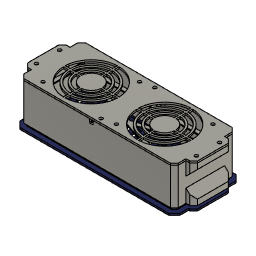
Exhaust (Autodesk Fusion 360 archive; units mm, degrees)
design "Exhaust Fan Cover"
Autodesk Fusion 360 part; units mm, degrees
(part 1 of 2)
sketch "Skizze1" plane through (0, 0, 0) normal (0, 0, 1) x (1, 0, 0)
  line L0 (0, 0) -> (160, 0)
  line L1 (160, 0) -> (160, 64)
  line L2 (160, 64) -> (0, 64)
  line L3 (0, 64) -> (0, 0)
  dimension "d1" = 160
  dimension "d2" = 64
  constraint horizontal L0
  constraint vertical L1
  constraint horizontal L2
  constraint vertical L3
  constraint coincident L0.start L3.end
  measures "d1" distance of L0.start L0.end
  measures "d2" distance of L0.start L2.end
extrude "Extrusion1" add sketch "Skizze1" along normal blind 40 makes body 1
chamfer "Fase1" distance 4 angle 45 4 edges at (160, 0, 20) (160, 64, 20) (0, 0, 20) (0, 64, 20) on bodies 1
shell "Schale1" thickness 1.8 removed faces 1 at (54.6667, 42.6667, 40) on bodies 1
sketch "Skizze2" plane through (0, 0, 1.8) normal (0, 0, 1) x (-1, 0, 0)
  line L0 (-4.7456, -62.2) -> (-1.8, -59.2544)
  line L1 (-1.8, -59.2544) -> (-1.8, -4.7456)
  line L2 (-1.8, -4.7456) -> (-4.7456, -1.8)
  line L3 (-4.7456, -1.8) -> (-155.2544, -1.8)
  line L4 (-155.2544, -1.8) -> (-158.2, -4.7456)
  line L5 (-158.2, -4.7456) -> (-158.2, -59.2544)
  line L6 (-158.2, -59.2544) -> (-155.2544, -62.2)
  line L7 (-155.2544, -62.2) -> (-4.7456, -62.2)
  line L8 (-80, -57) -> (-80, -7) construction
  line L9 (-78, -7) -> (-69.1837, -57)
  line L10 (-69.1837, -57) -> (-65.1219, -57)
  line L11 (-65.1219, -57) -> (-73.9383, -7)
  line L12 (-73.9383, -7) -> (-78, -7)
  line L13 (-56.8362, -57) -> (-65.6526, -7)
  line L14 (-69.7143, -7) -> (-60.8979, -57)
  line L15 (-60.8979, -57) -> (-56.8362, -57)
  line L16 (-65.6526, -7) -> (-69.7143, -7)
  line L17 (-48.5505, -57) -> (-57.3669, -7)
  line L18 (-61.4286, -7) -> (-52.6122, -57)
  line L19 (-52.6122, -57) -> (-48.5505, -57)
  line L20 (-57.3669, -7) -> (-61.4286, -7)
  line L21 (-40.2648, -57) -> (-49.0812, -7)
  line L22 (-53.1429, -7) -> (-44.3265, -57)
  line L23 (-44.3265, -57) -> (-40.2648, -57)
  line L24 (-49.0812, -7) -> (-53.1429, -7)
  line L25 (-31.9791, -57) -> (-40.7954, -7)
  line L26 (-44.8571, -7) -> (-36.0408, -57)
  line L27 (-36.0408, -57) -> (-31.9791, -57)
  line L28 (-40.7954, -7) -> (-44.8571, -7)
  line L29 (-23.6934, -57) -> (-32.5097, -7)
  line L30 (-36.5714, -7) -> (-27.7551, -57)
  line L31 (-27.7551, -57) -> (-23.6934, -57)
  line L32 (-32.5097, -7) -> (-36.5714, -7)
  line L33 (-15.4077, -57) -> (-24.224, -7)
  line L34 (-28.2857, -7) -> (-19.4694, -57)
  line L35 (-19.4694, -57) -> (-15.4077, -57)
  line L36 (-24.224, -7) -> (-28.2857, -7)
  line L37 (-7.1219, -57) -> (-15.9383, -7)
  line L38 (-20, -7) -> (-11.1837, -57)
  line L39 (-11.1837, -57) -> (-7.1219, -57)
  line L40 (-15.9383, -7) -> (-20, -7)
  line L41 (-11.7183, -7) -> (-8, -28.0875)
  line L42 (-11.7183, -7) -> (13.942, -7) construction
  line L43 (-8, -28.0875) -> (-7, -28.0875)
  line L44 (-7, -10.7237) -> (-7.6566, -7)
  line L45 (-7.6566, -7) -> (-11.7183, -7)
  line L46 (-7, -28.0875) -> (-7, -10.7237)
  line L47 (-119.7352, -57) -> (-110.9188, -7)
  line L48 (-153, -28.0875) -> (-153, -10.7237)
  line L49 (-152, -28.0875) -> (-153, -28.0875)
  line L50 (-98.5714, -7) -> (-107.3878, -57)
  line L51 (-152.3434, -7) -> (-148.2817, -7)
  line L52 (-119.2046, -7) -> (-115.1429, -7)
  line L53 (-132.2449, -57) -> (-136.3066, -57)
  line L54 (-135.776, -7) -> (-131.7143, -7)
  line L55 (-140.5306, -57) -> (-144.5923, -57)
  line L56 (-102.6331, -7) -> (-98.5714, -7)
  line L57 (-153, -10.7237) -> (-152.3434, -7)
  line L58 (-99.1021, -57) -> (-103.1638, -57)
  line L59 (-106.8571, -7) -> (-115.6735, -57)
  line L60 (-107.3878, -57) -> (-111.4495, -57)
  line L61 (-123.9592, -57) -> (-128.0209, -57)
  line L62 (-115.6735, -57) -> (-119.7352, -57)
  line L63 (-128.0209, -57) -> (-119.2046, -7)
  line L64 (-144.5923, -57) -> (-135.776, -7)
  line L65 (-111.4495, -57) -> (-102.6331, -7)
  line L66 (-131.7143, -7) -> (-140.5306, -57)
  line L67 (-148.8163, -57) -> (-152.8781, -57)
  line L68 (-123.4286, -7) -> (-132.2449, -57)
  line L69 (-140, -7) -> (-148.8163, -57)
  line L70 (-148.2817, -7) -> (-152, -28.0875)
  line L71 (-115.1429, -7) -> (-123.9592, -57)
  line L72 (-127.4903, -7) -> (-123.4286, -7)
  line L73 (-144.0617, -7) -> (-140, -7)
  line L74 (-90.8163, -57) -> (-94.8781, -57)
  line L75 (-90.2857, -7) -> (-99.1021, -57)
  line L76 (-82, -7) -> (-90.8163, -57)
  line L77 (-86.0617, -7) -> (-82, -7)
  line L78 (-103.1638, -57) -> (-94.3474, -7)
  line L79 (-94.3474, -7) -> (-90.2857, -7)
  line L80 (-110.9188, -7) -> (-106.8571, -7)
  line L81 (-94.8781, -57) -> (-86.0617, -7)
  line L82 (-136.3066, -57) -> (-127.4903, -7)
  line L83 (-152.8781, -57) -> (-144.0617, -7)
  line L84 (-78.7624, -26.609) -> (-73.4037, -57)
  line L85 (-73.4037, -57) -> (-77.4654, -57)
  line L86 (-77.4654, -57) -> (-79.1, -47.7295)
  line L87 (-79.1, -47.7295) -> (-80, -47.7295)
  line L88 (-78.7624, -26.609) -> (-80, -26.609)
  line L89 (-82.5346, -57) -> (-80.9, -47.7295)
  line L90 (-86.5963, -57) -> (-82.5346, -57)
  line L91 (-81.2376, -26.609) -> (-86.5963, -57)
  line L92 (-81.2376, -26.609) -> (-80, -26.609)
  line L93 (-80.9, -47.7295) -> (-80, -47.7295)
  line L94 (-7, -57) -> (-7, -7) construction
  line L95 (-7, -7) -> (-153, -7) construction
  line L96 (-153, -7) -> (-153, -57) construction
  line L97 (-153, -57) -> (-7, -57) construction
  point P0 (-80, -57)
  point P1 (-80, -7)
  dimension "d7" = -5.2
  dimension "d8" = 4
  dimension "d9" = 80
  dimension "d10" = 2
  dimension "d13" = 58
  dimension "d14" = 0
  dimension "d15" = 80
  dimension "d16" = 4
  dimension "d17" = 4.22
  dimension "d18" = 1
  dimension "d19" = 4
  dimension "d20" = 0.9
  dimension "d21" = 4.22
  constraint midpoint P0 L97
  constraint midpoint P1 L95
  constraint coincident L9.start L95
  constraint coincident L9.end L97
  constraint coincident L10.end L97
  constraint coincident L11.end L95
  constraint parallel L9 L11
  constraint horizontal L42
  constraint coincident L41.start L95
  constraint coincident L44.start L94
  constraint perpendicular L43 L94
  constraint parallel L41 L44
  constraint coincident L44.end L95
  constraint coincident L43.end L94
  constraint symmetric P0 L8 L8.start
  constraint symmetric P1 L8 L8.end
  constraint symmetric L8 L9.start L76.start
  constraint symmetric L8 L9.end L74.start
  constraint symmetric L8 L10.end L74.end
  constraint symmetric L8 L11.end L77.start
  constraint symmetric L8 L13.start L58.end
  constraint symmetric L8 L13.end L78.end
  constraint symmetric L8 L14.start L75.start
  constraint symmetric L8 L14.end L58.start
  constraint symmetric L8 L17.start L60.end
  constraint symmetric L8 L17.end L56.start
  constraint symmetric L8 L18.start L50.start
  constraint symmetric L8 L18.end L50.end
  constraint symmetric L8 L21.start L47.start
  constraint symmetric L8 L21.end L47.end
  constraint symmetric L8 L22.start L59.start
  constraint symmetric L8 L22.end L59.end
  constraint symmetric L8 L25.start L61.end
  constraint symmetric L8 L25.end L52.start
  constraint symmetric L8 L26.start L52.end
  constraint symmetric L8 L26.end L61.start
  constraint symmetric L8 L29.start L53.end
  constraint symmetric L8 L29.end L72.start
  constraint symmetric L8 L30.start L68.start
  constraint symmetric L8 L30.end L53.start
  constraint symmetric L8 L33.start L55.end
  constraint symmetric L8 L33.end L54.start
  constraint symmetric L8 L34.start L54.end
  constraint symmetric L8 L34.end L55.start
  constraint symmetric L8 L37.start L67.end
  constraint symmetric L8 L37.end L73.start
  constraint symmetric L8 L38.start L69.start
  constraint symmetric L8 L38.end L67.start
  constraint symmetric L8 L41.start L51.end
  constraint symmetric L8 L41.end L49.start
  constraint symmetric L8 L44.start L48.end
  constraint symmetric L8 L44.end L51.start
  constraint symmetric L8 L43.end L48.start
  constraint coincident L84.end L97
  constraint parallel L9 L84
  constraint coincident L85.end L97
  constraint parallel L84 L86
  constraint coincident L8 L87.end
  constraint perpendicular L8 L87
  constraint coincident L8 L88.end
  constraint perpendicular L8 L88
  constraint symmetric L8 L84.start L91.start
  constraint symmetric L8 L84.end L90.start
  constraint symmetric L8 L85.end L89.start
  constraint symmetric L8 L86.end L89.end
  constraint symmetric L8 L87.end L93.end
  constraint symmetric L8 L88.end L92.end
  measures "d8" distance of L9 L11
  measures "d9" angle of L11 L95
  measures "d10" distance of P1 L9.start
  measures "d15" angle of L41 L42
  measures "d16" distance of L41 L44
  measures "d17" distance of L37.end L41.start
  measures "d18" distance of L41.end L43.end
  measures "d19" distance of L84 L86
  measures "d20" distance of L86.end L87.end
  measures "d21" distance of L9.end L84.end
extrude "Extrusion2" cut sketch "Skizze2" against normal blind 1.8 contours L9 L10 L11 L12 | L13 L14 L15 L16 | L17 L18 L19 L20 | L21 L22 L23 L24 | L25 L26 L27 L28 | L29 L30 L31 L32 | L33 L34 L35 L36 | L37 L38 L39 L40 | L41 L43 L44 L45 L46 | L47 L59 L62 L80 | L48 L49 L51 L57 L70 | L50 L56 L60 L65 | L52 L61 L63 L71 | L53 L68 L72 L82 | L54 L55 L64 L66 | L58 L75 L78 L79 | L67 L69 L73 L83 | L74 L76 L77 L81 | L84 L85 L86 L87 L88 L89 L90 L91 L92 L93 bodies 1
ref_plane "Arbeitsebene1" through (80, 32, 1.8) normal (0, 0, -1) x (-1, 0, 0)
split "Teilen1" by plane through (80, 32, 1.8) normal (0, 0, -1) bodies 1 makes body 2 at (80.6667, 2.3333, 0)
sketch "Skizze3" plane through (0, 0, 1.8) normal (0, 0, -1) x (1, 0, 0)
  line L0 (158.2, -59.2544) -> (155.2544, -62.2)
  line L1 (155.2544, -62.2) -> (4.7456, -62.2)
  line L2 (4.7456, -62.2) -> (1.8, -59.2544)
  line L3 (1.8, -59.2544) -> (1.8, -4.7456)
  line L4 (1.8, -4.7456) -> (4.7456, -1.8)
  line L5 (4.7456, -1.8) -> (155.2544, -1.8)
  line L6 (155.2544, -1.8) -> (158.2, -4.7456)
  line L7 (158.2, -4.7456) -> (158.2, -59.2544)
  line L8 (156, -64) -> (160, -60)
  line L9 (160, -60) -> (160, -4)
  line L10 (160, -4) -> (156, 0)
  line L11 (156, 0) -> (4, 0)
  line L12 (4, 0) -> (0, -4)
  line L13 (0, -4) -> (0, -60)
  line L14 (0, -60) -> (4, -64)
  line L15 (4, -64) -> (156, -64)
  line L16 (80, -1.8) -> (80, -62.2) construction
  line L17 (0, -12) -> (-8, -12)
  line L18 (-8, -12) -> (-8, -52)
  line L19 (-8, -52) -> (0, -52)
  line L20 (0, -52) -> (0, -12)
  line L21 (80, -32) -> (1.8, -32) construction
  line L22 (160, -12) -> (168, -12)
  line L23 (168, -12) -> (168, -52)
  line L24 (168, -52) -> (160, -52)
  dimension "d25" = 40
  dimension "d26" = 8
  constraint midpoint L5 L16.start
  constraint midpoint L1 L16.end
  constraint horizontal L17
  constraint vertical L18
  constraint horizontal L19
  constraint vertical L20
  constraint coincident L13 L17.start
  constraint midpoint L16 L21.start
  constraint midpoint L3 L21.end
  constraint symmetric L17 L19 L21
  constraint symmetric L16 L17.start L22.start
  constraint symmetric L16 L17.end L22.end
  constraint symmetric L16 L18.end L23.end
  constraint symmetric L16 L19.end L24.end
  measures "d25" distance of L17.end L18.end
  measures "d26" distance of L17.start L17.end
extrude "Extrusion3" add sketch "Skizze3" against normal blind 5.8 contours L9 L22 L23 L24 | L13 L17 L18 L19 L20 bodies 1 2
chamfer "Fase2" distance 4 angle 45 4 edges at (168, 52, 4.7) (168, 12, 4.7) (-8, 52, 4.7) (-8, 12, 4.7) on bodies 1
sketch "Skizze4" plane through (0, 0, 0) normal (0, 0, -1) x (1, 0, 0)
  line L0 (135.776, -7) -> (144.5923, -57)
  line L1 (144.5923, -57) -> (140.5306, -57)
  line L2 (140.5306, -57) -> (131.7143, -7)
  line L3 (131.7143, -7) -> (135.776, -7)
  line L4 (107.3878, -57) -> (98.5714, -7)
  line L5 (98.5714, -7) -> (102.6331, -7)
  line L6 (102.6331, -7) -> (111.4495, -57)
  line L7 (111.4495, -57) -> (107.3878, -57)
  line L8 (78, -7) -> (69.1837, -57)
  line L9 (69.1837, -57) -> (65.1219, -57)
  line L10 (65.1219, -57) -> (73.9383, -7)
  line L11 (73.9383, -7) -> (78, -7)
  line L12 (44.8571, -7) -> (36.0408, -57)
  line L13 (36.0408, -57) -> (31.9791, -57)
  line L14 (31.9791, -57) -> (40.7954, -7)
  line L15 (40.7954, -7) -> (44.8571, -7)
  line L16 (7, -10.7237) -> (7.6566, -7)
  line L17 (7.6566, -7) -> (11.7183, -7)
  line L18 (11.7183, -7) -> (8, -28.0875)
  line L19 (8, -28.0875) -> (7, -28.0875)
  line L20 (7, -28.0875) -> (7, -10.7237)
  line L21 (36.5714, -7) -> (27.7551, -57)
  line L22 (27.7551, -57) -> (23.6934, -57)
  line L23 (23.6934, -57) -> (32.5097, -7)
  line L24 (32.5097, -7) -> (36.5714, -7)
  line L25 (69.7143, -7) -> (60.8979, -57)
  line L26 (60.8979, -57) -> (56.8362, -57)
  line L27 (56.8362, -57) -> (65.6526, -7)
  line L28 (65.6526, -7) -> (69.7143, -7)
  line L29 (103.1638, -57) -> (99.1021, -57)
  line L30 (99.1021, -57) -> (90.2857, -7)
  line L31 (90.2857, -7) -> (94.3474, -7)
  line L32 (94.3474, -7) -> (103.1638, -57)
  line L33 (132.2449, -57) -> (123.4286, -7)
  line L34 (123.4286, -7) -> (127.4903, -7)
  line L35 (127.4903, -7) -> (136.3066, -57)
  line L36 (136.3066, -57) -> (132.2449, -57)
  line L37 (148.8163, -57) -> (140, -7)
  line L38 (140, -7) -> (144.0617, -7)
  line L39 (144.0617, -7) -> (152.8781, -57)
  line L40 (152.8781, -57) -> (148.8163, -57)
  line L41 (119.7352, -57) -> (115.6735, -57)
  line L42 (115.6735, -57) -> (106.8571, -7)
  line L43 (106.8571, -7) -> (110.9188, -7)
  line L44 (110.9188, -7) -> (119.7352, -57)
  line L45 (86.5963, -57) -> (82.5346, -57)
  line L46 (82.5346, -57) -> (80.9, -47.7295)
  line L47 (80.9, -47.7295) -> (79.1, -47.7295)
  line L48 (79.1, -47.7295) -> (77.4654, -57)
  line L49 (77.4654, -57) -> (73.4037, -57)
  line L50 (73.4037, -57) -> (78.7624, -26.609)
  line L51 (78.7624, -26.609) -> (81.2376, -26.609)
  line L52 (81.2376, -26.609) -> (86.5963, -57)
  line L53 (53.1429, -7) -> (44.3265, -57)
  line L54 (44.3265, -57) -> (40.2648, -57)
  line L55 (40.2648, -57) -> (49.0812, -7)
  line L56 (49.0812, -7) -> (53.1429, -7)
  line L57 (20, -7) -> (11.1837, -57)
  line L58 (11.1837, -57) -> (7.1219, -57)
  line L59 (7.1219, -57) -> (15.9383, -7)
  line L60 (15.9383, -7) -> (20, -7)
  line L61 (28.2857, -7) -> (19.4694, -57)
  line L62 (19.4694, -57) -> (15.4077, -57)
  line L63 (15.4077, -57) -> (24.224, -7)
  line L64 (24.224, -7) -> (28.2857, -7)
  line L65 (61.4286, -7) -> (52.6122, -57)
  line L66 (52.6122, -57) -> (48.5505, -57)
  line L67 (48.5505, -57) -> (57.3669, -7)
  line L68 (57.3669, -7) -> (61.4286, -7)
  line L69 (90.8163, -57) -> (82, -7)
  line L70 (82, -7) -> (86.0617, -7)
  line L71 (86.0617, -7) -> (94.8781, -57)
  line L72 (94.8781, -57) -> (90.8163, -57)
  line L73 (119.2046, -7) -> (128.0209, -57)
  line L74 (128.0209, -57) -> (123.9592, -57)
  line L75 (123.9592, -57) -> (115.1429, -7)
  line L76 (115.1429, -7) -> (119.2046, -7)
  line L77 (152.3434, -7) -> (153, -10.7237)
  line L78 (153, -10.7237) -> (153, -28.0875)
  line L79 (153, -28.0875) -> (152, -28.0875)
  line L80 (152, -28.0875) -> (148.2817, -7)
  line L81 (148.2817, -7) -> (152.3434, -7)
  line L82 (0, -60) -> (4, -64)
  line L83 (4, -64) -> (156, -64)
  line L84 (156, -64) -> (160, -60)
  line L85 (160, -60) -> (160, -4)
  line L86 (160, -4) -> (156, 0)
  line L87 (156, 0) -> (4, 0)
  line L88 (4, 0) -> (0, -4)
  line L89 (0, -4) -> (0, -60)
  line L90 (162.8, -61.1598) -> (162.8, -2.8402)
  line L91 (162.8, -2.8402) -> (157.1598, 2.8)
  line L92 (157.1598, 2.8) -> (2.8402, 2.8)
  line L93 (2.8402, 2.8) -> (-2.8, -2.8402)
  line L94 (-2.8, -2.8402) -> (-2.8, -61.1598)
  line L95 (-2.8, -61.1598) -> (2.8402, -66.8)
  line L96 (2.8402, -66.8) -> (157.1598, -66.8)
  line L97 (157.1598, -66.8) -> (162.8, -61.1598)
  dimension "d30" = 2.8
extrude "Extrusion4" add sketch "Skizze4" against normal blind 1.8 contours L90 L91 L92 L93 L94 L95 L96 L97 bodies 1
sketch "Skizze5" plane through (0, 0, 1.8) normal (0, 0, 1) x (-1, 0, 0)
  line L0 (-144.5923, -57) -> (-135.776, -7)
  line L1 (-135.776, -7) -> (-131.7143, -7)
  line L2 (-131.7143, -7) -> (-140.5306, -57)
  line L3 (-140.5306, -57) -> (-144.5923, -57)
  line L4 (-98.5714, -7) -> (-107.3878, -57)
  line L5 (-107.3878, -57) -> (-111.4495, -57)
  line L6 (-111.4495, -57) -> (-102.6331, -7)
  line L7 (-102.6331, -7) -> (-98.5714, -7)
  line L8 (-69.1837, -57) -> (-78, -7)
  line L9 (-78, -7) -> (-73.9383, -7)
  line L10 (-73.9383, -7) -> (-65.1219, -57)
  line L11 (-65.1219, -57) -> (-69.1837, -57)
  line L12 (-36.0408, -57) -> (-44.8571, -7)
  line L13 (-44.8571, -7) -> (-40.7954, -7)
  line L14 (-40.7954, -7) -> (-31.9791, -57)
  line L15 (-31.9791, -57) -> (-36.0408, -57)
  line L16 (-7.6566, -7) -> (-7, -10.7237)
  line L17 (-7, -10.7237) -> (-7, -28.0875)
  line L18 (-7, -28.0875) -> (-8, -28.0875)
  line L19 (-8, -28.0875) -> (-11.7183, -7)
  line L20 (-11.7183, -7) -> (-7.6566, -7)
  line L21 (-27.7551, -57) -> (-36.5714, -7)
  line L22 (-36.5714, -7) -> (-32.5097, -7)
  line L23 (-32.5097, -7) -> (-23.6934, -57)
  line L24 (-23.6934, -57) -> (-27.7551, -57)
  line L25 (-60.8979, -57) -> (-69.7143, -7)
  line L26 (-69.7143, -7) -> (-65.6526, -7)
  line L27 (-65.6526, -7) -> (-56.8362, -57)
  line L28 (-56.8362, -57) -> (-60.8979, -57)
  line L29 (-99.1021, -57) -> (-103.1638, -57)
  line L30 (-103.1638, -57) -> (-94.3474, -7)
  line L31 (-94.3474, -7) -> (-90.2857, -7)
  line L32 (-90.2857, -7) -> (-99.1021, -57)
  line L33 (-123.4286, -7) -> (-132.2449, -57)
  line L34 (-132.2449, -57) -> (-136.3066, -57)
  line L35 (-136.3066, -57) -> (-127.4903, -7)
  line L36 (-127.4903, -7) -> (-123.4286, -7)
  line L37 (-140, -7) -> (-148.8163, -57)
  line L38 (-148.8163, -57) -> (-152.8781, -57)
  line L39 (-152.8781, -57) -> (-144.0617, -7)
  line L40 (-144.0617, -7) -> (-140, -7)
  line L41 (-115.6735, -57) -> (-119.7352, -57)
  line L42 (-119.7352, -57) -> (-110.9188, -7)
  line L43 (-110.9188, -7) -> (-106.8571, -7)
  line L44 (-106.8571, -7) -> (-115.6735, -57)
  line L45 (-82.5346, -57) -> (-86.5963, -57)
  line L46 (-86.5963, -57) -> (-81.2376, -26.609)
  line L47 (-81.2376, -26.609) -> (-78.7624, -26.609)
  line L48 (-78.7624, -26.609) -> (-73.4037, -57)
  line L49 (-73.4037, -57) -> (-77.4654, -57)
  line L50 (-77.4654, -57) -> (-79.1, -47.7295)
  line L51 (-79.1, -47.7295) -> (-80.9, -47.7295)
  line L52 (-80.9, -47.7295) -> (-82.5346, -57)
  line L53 (-44.3265, -57) -> (-53.1429, -7)
  line L54 (-53.1429, -7) -> (-49.0812, -7)
  line L55 (-49.0812, -7) -> (-40.2648, -57)
  line L56 (-40.2648, -57) -> (-44.3265, -57)
  line L57 (-11.1837, -57) -> (-20, -7)
  line L58 (-20, -7) -> (-15.9383, -7)
  line L59 (-15.9383, -7) -> (-7.1219, -57)
  line L60 (-7.1219, -57) -> (-11.1837, -57)
  line L61 (-19.4694, -57) -> (-28.2857, -7)
  line L62 (-28.2857, -7) -> (-24.224, -7)
  line L63 (-24.224, -7) -> (-15.4077, -57)
  line L64 (-15.4077, -57) -> (-19.4694, -57)
  line L65 (-52.6122, -57) -> (-61.4286, -7)
  line L66 (-61.4286, -7) -> (-57.3669, -7)
  line L67 (-57.3669, -7) -> (-48.5505, -57)
  line L68 (-48.5505, -57) -> (-52.6122, -57)
  line L69 (-82, -7) -> (-90.8163, -57)
  line L70 (-90.8163, -57) -> (-94.8781, -57)
  line L71 (-94.8781, -57) -> (-86.0617, -7)
  line L72 (-86.0617, -7) -> (-82, -7)
  line L73 (-128.0209, -57) -> (-119.2046, -7)
  line L74 (-119.2046, -7) -> (-115.1429, -7)
  line L75 (-115.1429, -7) -> (-123.9592, -57)
  line L76 (-123.9592, -57) -> (-128.0209, -57)
  line L77 (-153, -10.7237) -> (-152.3434, -7)
  line L78 (-152.3434, -7) -> (-148.2817, -7)
  line L79 (-148.2817, -7) -> (-152, -28.0875)
  line L80 (-152, -28.0875) -> (-153, -28.0875)
  line L81 (-153, -28.0875) -> (-153, -10.7237)
  line L82 (-2, -59.1716) -> (-2, -4.8284)
  line L83 (-2, -4.8284) -> (-4.8284, -2)
  line L84 (-4.8284, -2) -> (-155.1716, -2)
  line L85 (-155.1716, -2) -> (-158, -4.8284)
  line L86 (-158, -4.8284) -> (-158, -59.1716)
  line L87 (-158, -59.1716) -> (-155.1716, -62)
  line L88 (-155.1716, -62) -> (-4.8284, -62)
  line L89 (-4.8284, -62) -> (-2, -59.1716)
  line L90 (-3.8, -58.426) -> (-3.8, -5.574)
  line L91 (-3.8, -5.574) -> (-5.574, -3.8)
  line L92 (-5.574, -3.8) -> (-154.426, -3.8)
  line L93 (-154.426, -3.8) -> (-156.2, -5.574)
  line L94 (-156.2, -5.574) -> (-156.2, -58.426)
  line L95 (-156.2, -58.426) -> (-154.426, -60.2)
  line L96 (-154.426, -60.2) -> (-5.574, -60.2)
  line L97 (-5.574, -60.2) -> (-3.8, -58.426)
  line L98 (-155.2544, -62.2) -> (-4.7456, -62.2)
  line L99 (-4.7456, -62.2) -> (-1.8, -59.2544)
  line L100 (-1.8, -59.2544) -> (-1.8, -4.7456)
  line L101 (-1.8, -4.7456) -> (-4.7456, -1.8)
  line L102 (-4.7456, -1.8) -> (-155.2544, -1.8)
  line L103 (-155.2544, -1.8) -> (-158.2, -4.7456)
  line L104 (-158.2, -4.7456) -> (-158.2, -59.2544)
  line L105 (-158.2, -59.2544) -> (-155.2544, -62.2)
extrude "Extrusion5" add sketch "Skizze5" along normal blind 4 contours L82 L83 L84 L85 L86 L87 L88 L89 bodies 1
sketch "Skizze6" plane through (0, 0, 0) normal (0, 0, -1) x (1, 0, 0)
  line L0 (157.1598, -66.8) -> (162.8, -61.1598)
  line L1 (162.8, -61.1598) -> (162.8, -2.8402)
  line L2 (162.8, -2.8402) -> (157.1598, 2.8)
  line L3 (157.1598, 2.8) -> (2.8402, 2.8)
  line L4 (2.8402, 2.8) -> (-2.8, -2.8402)
  line L5 (-2.8, -2.8402) -> (-2.8, -61.1598)
  line L6 (-2.8, -61.1598) -> (2.8402, -66.8)
  line L7 (2.8402, -66.8) -> (157.1598, -66.8)
  line L8 (135.776, -7) -> (144.5923, -57)
  line L9 (144.5923, -57) -> (140.5306, -57)
  line L10 (140.5306, -57) -> (131.7143, -7)
  line L11 (131.7143, -7) -> (135.776, -7)
  line L12 (107.3878, -57) -> (98.5714, -7)
  line L13 (98.5714, -7) -> (102.6331, -7)
  line L14 (102.6331, -7) -> (111.4495, -57)
  line L15 (111.4495, -57) -> (107.3878, -57)
  line L16 (78, -7) -> (69.1837, -57)
  line L17 (69.1837, -57) -> (65.1219, -57)
  line L18 (65.1219, -57) -> (73.9383, -7)
  line L19 (73.9383, -7) -> (78, -7)
  line L20 (44.8571, -7) -> (36.0408, -57)
  line L21 (36.0408, -57) -> (31.9791, -57)
  line L22 (31.9791, -57) -> (40.7954, -7)
  line L23 (40.7954, -7) -> (44.8571, -7)
  line L24 (7, -10.7237) -> (7.6566, -7)
  line L25 (7.6566, -7) -> (11.7183, -7)
  line L26 (11.7183, -7) -> (8, -28.0875)
  line L27 (8, -28.0875) -> (7, -28.0875)
  line L28 (7, -28.0875) -> (7, -10.7237)
  line L29 (36.5714, -7) -> (27.7551, -57)
  line L30 (27.7551, -57) -> (23.6934, -57)
  line L31 (23.6934, -57) -> (32.5097, -7)
  line L32 (32.5097, -7) -> (36.5714, -7)
  line L33 (69.7143, -7) -> (60.8979, -57)
  line L34 (60.8979, -57) -> (56.8362, -57)
  line L35 (56.8362, -57) -> (65.6526, -7)
  line L36 (65.6526, -7) -> (69.7143, -7)
  line L37 (103.1638, -57) -> (99.1021, -57)
  line L38 (99.1021, -57) -> (90.2857, -7)
  line L39 (90.2857, -7) -> (94.3474, -7)
  line L40 (94.3474, -7) -> (103.1638, -57)
  line L41 (132.2449, -57) -> (123.4286, -7)
  line L42 (123.4286, -7) -> (127.4903, -7)
  line L43 (127.4903, -7) -> (136.3066, -57)
  line L44 (136.3066, -57) -> (132.2449, -57)
  line L45 (148.8163, -57) -> (140, -7)
  line L46 (140, -7) -> (144.0617, -7)
  line L47 (144.0617, -7) -> (152.8781, -57)
  line L48 (152.8781, -57) -> (148.8163, -57)
  line L49 (119.7352, -57) -> (115.6735, -57)
  line L50 (115.6735, -57) -> (106.8571, -7)
  line L51 (106.8571, -7) -> (110.9188, -7)
  line L52 (110.9188, -7) -> (119.7352, -57)
  line L53 (86.5963, -57) -> (82.5346, -57)
  line L54 (82.5346, -57) -> (80.9, -47.7295)
  line L55 (80.9, -47.7295) -> (79.1, -47.7295)
  line L56 (79.1, -47.7295) -> (77.4654, -57)
  line L57 (77.4654, -57) -> (73.4037, -57)
  line L58 (73.4037, -57) -> (78.7624, -26.609)
  line L59 (78.7624, -26.609) -> (81.2376, -26.609)
  line L60 (81.2376, -26.609) -> (86.5963, -57)
  line L61 (53.1429, -7) -> (44.3265, -57)
  line L62 (44.3265, -57) -> (40.2648, -57)
  line L63 (40.2648, -57) -> (49.0812, -7)
  line L64 (49.0812, -7) -> (53.1429, -7)
  line L65 (20, -7) -> (11.1837, -57)
  line L66 (11.1837, -57) -> (7.1219, -57)
  line L67 (7.1219, -57) -> (15.9383, -7)
  line L68 (15.9383, -7) -> (20, -7)
  line L69 (28.2857, -7) -> (19.4694, -57)
  line L70 (19.4694, -57) -> (15.4077, -57)
  line L71 (15.4077, -57) -> (24.224, -7)
  line L72 (24.224, -7) -> (28.2857, -7)
  line L73 (61.4286, -7) -> (52.6122, -57)
  line L74 (52.6122, -57) -> (48.5505, -57)
  line L75 (48.5505, -57) -> (57.3669, -7)
  line L76 (57.3669, -7) -> (61.4286, -7)
  line L77 (90.8163, -57) -> (82, -7)
  line L78 (82, -7) -> (86.0617, -7)
  line L79 (86.0617, -7) -> (94.8781, -57)
  line L80 (94.8781, -57) -> (90.8163, -57)
  line L81 (119.2046, -7) -> (128.0209, -57)
  line L82 (128.0209, -57) -> (123.9592, -57)
  line L83 (123.9592, -57) -> (115.1429, -7)
  line L84 (115.1429, -7) -> (119.2046, -7)
  line L85 (152.3434, -7) -> (153, -10.7237)
  line L86 (153, -10.7237) -> (153, -28.0875)
  line L87 (153, -28.0875) -> (152, -28.0875)
  line L88 (152, -28.0875) -> (148.2817, -7)
  line L89 (148.2817, -7) -> (152.3434, -7)
  line L90 (-8, -16) -> (-4, -12)
  line L91 (-2.8, -12) -> (-4, -12)
  line L92 (-8, -16) -> (-8, -48)
  line L93 (-4, -52) -> (-8, -48)
  line L94 (-4, -52) -> (-2.8, -52)
  line L95 (162.8, -12) -> (164, -12)
  line L96 (164, -12) -> (168, -16)
  line L97 (168, -16) -> (168, -48)
  line L98 (168, -48) -> (164, -52)
  line L99 (164, -52) -> (162.8, -52)
  point P0 (162.8, -52)
  point P1 (164, -52)
extrude "Extrusion6" add sketch "Skizze6" against normal blind 1.8 contours L1 L95 L96 L97 L98 L99 | L5 L90 L91 L92 L93 L94 bodies 1
ref_plane "Arbeitsebene2" through (80, 4.6, 1.8) normal (0, 0, 1) x (1, 0, 0)
split "Teilen2" by plane through (80, 4.6, 1.8) normal (0, 0, 1) bodies 1 makes body 3 at (105.3333, 64, 14.5333) makes body 4 at (104.8087, 2.6, 5.8)
combine "Kombinieren1" operation add target body 4 tool bodies 1
move_body "Verschieben2" bodies 4 to x (1, 0, 0) y (0, 1, 0) z (0, 0, 1) at (0, 0, -3)
sketch "Skizze7" plane through (0, 0, -3) normal (0, 0, -1) x (1, 0, 0)
  line L0 (157.1598, -66.8) -> (162.8, -61.1598)
  line L1 (162.8, -61.1598) -> (162.8, -52)
  line L2 (162.8, -52) -> (164, -52)
  line L3 (164, -52) -> (168, -48)
  line L4 (168, -48) -> (168, -16)
  line L5 (168, -16) -> (164, -12)
  line L6 (164, -12) -> (162.8, -12)
  line L7 (162.8, -12) -> (162.8, -2.8402)
  line L8 (162.8, -2.8402) -> (157.1598, 2.8)
  line L9 (157.1598, 2.8) -> (2.8402, 2.8)
  line L10 (2.8402, 2.8) -> (-2.8, -2.8402)
  line L11 (-2.8, -2.8402) -> (-2.8, -12)
  line L12 (-2.8, -12) -> (-4, -12)
  line L13 (-4, -12) -> (-8, -16)
  line L14 (-8, -16) -> (-8, -48)
  line L15 (-8, -48) -> (-4, -52)
  line L16 (-4, -52) -> (-2.8, -52)
  line L17 (-2.8, -52) -> (-2.8, -61.1598)
  line L18 (-2.8, -61.1598) -> (2.8402, -66.8)
  line L19 (2.8402, -66.8) -> (157.1598, -66.8)
  line L20 (135.776, -7) -> (144.5923, -57)
  line L21 (144.5923, -57) -> (140.5306, -57)
  line L22 (140.5306, -57) -> (131.7143, -7)
  line L23 (131.7143, -7) -> (135.776, -7)
  line L24 (107.3878, -57) -> (98.5714, -7)
  line L25 (98.5714, -7) -> (102.6331, -7)
  line L26 (102.6331, -7) -> (111.4495, -57)
  line L27 (111.4495, -57) -> (107.3878, -57)
  line L28 (78, -7) -> (69.1837, -57)
  line L29 (69.1837, -57) -> (65.1219, -57)
  line L30 (65.1219, -57) -> (73.9383, -7)
  line L31 (73.9383, -7) -> (78, -7)
  line L32 (44.8571, -7) -> (36.0408, -57)
  line L33 (36.0408, -57) -> (31.9791, -57)
  line L34 (31.9791, -57) -> (40.7954, -7)
  line L35 (40.7954, -7) -> (44.8571, -7)
  line L36 (7, -10.7237) -> (7.6566, -7)
  line L37 (7.6566, -7) -> (11.7183, -7)
  line L38 (11.7183, -7) -> (8, -28.0875)
  line L39 (8, -28.0875) -> (7, -28.0875)
  line L40 (7, -28.0875) -> (7, -10.7237)
  line L41 (36.5714, -7) -> (27.7551, -57)
  line L42 (27.7551, -57) -> (23.6934, -57)
  line L43 (23.6934, -57) -> (32.5097, -7)
  line L44 (32.5097, -7) -> (36.5714, -7)
  line L45 (69.7143, -7) -> (60.8979, -57)
  line L46 (60.8979, -57) -> (56.8362, -57)
  line L47 (56.8362, -57) -> (65.6526, -7)
  line L48 (65.6526, -7) -> (69.7143, -7)
  line L49 (103.1638, -57) -> (99.1021, -57)
  line L50 (99.1021, -57) -> (90.2857, -7)
  line L51 (90.2857, -7) -> (94.3474, -7)
  line L52 (94.3474, -7) -> (103.1638, -57)
  line L53 (132.2449, -57) -> (123.4286, -7)
  line L54 (123.4286, -7) -> (127.4903, -7)
  line L55 (127.4903, -7) -> (136.3066, -57)
  line L56 (136.3066, -57) -> (132.2449, -57)
  line L57 (148.8163, -57) -> (140, -7)
  line L58 (140, -7) -> (144.0617, -7)
  line L59 (144.0617, -7) -> (152.8781, -57)
  line L60 (152.8781, -57) -> (148.8163, -57)
  line L61 (119.7352, -57) -> (115.6735, -57)
  line L62 (115.6735, -57) -> (106.8571, -7)
  line L63 (106.8571, -7) -> (110.9188, -7)
  line L64 (110.9188, -7) -> (119.7352, -57)
  line L65 (86.5963, -57) -> (82.5346, -57)
  line L66 (82.5346, -57) -> (80.9, -47.7295)
  line L67 (80.9, -47.7295) -> (79.1, -47.7295)
  line L68 (79.1, -47.7295) -> (77.4654, -57)
  line L69 (77.4654, -57) -> (73.4037, -57)
  line L70 (73.4037, -57) -> (78.7624, -26.609)
  line L71 (78.7624, -26.609) -> (81.2376, -26.609)
  line L72 (81.2376, -26.609) -> (86.5963, -57)
  line L73 (53.1429, -7) -> (44.3265, -57)
  line L74 (44.3265, -57) -> (40.2648, -57)
  line L75 (40.2648, -57) -> (49.0812, -7)
  line L76 (49.0812, -7) -> (53.1429, -7)
  line L77 (20, -7) -> (11.1837, -57)
  line L78 (11.1837, -57) -> (7.1219, -57)
  line L79 (7.1219, -57) -> (15.9383, -7)
  line L80 (15.9383, -7) -> (20, -7)
  line L81 (28.2857, -7) -> (19.4694, -57)
  line L82 (19.4694, -57) -> (15.4077, -57)
  line L83 (15.4077, -57) -> (24.224, -7)
  line L84 (24.224, -7) -> (28.2857, -7)
  line L85 (61.4286, -7) -> (52.6122, -57)
  line L86 (52.6122, -57) -> (48.5505, -57)
  line L87 (48.5505, -57) -> (57.3669, -7)
  line L88 (57.3669, -7) -> (61.4286, -7)
  line L89 (90.8163, -57) -> (82, -7)
  line L90 (82, -7) -> (86.0617, -7)
  line L91 (86.0617, -7) -> (94.8781, -57)
  line L92 (94.8781, -57) -> (90.8163, -57)
  line L93 (119.2046, -7) -> (128.0209, -57)
  line L94 (128.0209, -57) -> (123.9592, -57)
  line L95 (123.9592, -57) -> (115.1429, -7)
  line L96 (115.1429, -7) -> (119.2046, -7)
  line L97 (152.3434, -7) -> (153, -10.7237)
  line L98 (153, -10.7237) -> (153, -28.0875)
  line L99 (153, -28.0875) -> (152, -28.0875)
  line L100 (152, -28.0875) -> (148.2817, -7)
  line L101 (148.2817, -7) -> (152.3434, -7)
  line L102 (-2.8, -12) -> (-2.8, -52) construction
  line L103 (162.8, -12) -> (162.8, -52) construction
  circle A0 centre (162.8, -20) radius 1.7
  line L104 (162.8, -32) -> (-2.8, -32) construction
  line L105 (80, 2.8) -> (80, -66.8) construction
  circle A1 centre (162.8, -44) radius 1.7
  circle A2 centre (-2.8, -20) radius 1.7
  circle A3 centre (-2.8, -44) radius 1.7
  dimension "d40" = 3.4
  dimension "d41" = 24
  constraint coincident L11.end L12.start
  constraint coincident L16.end L17.start
  constraint coincident L6.end L7.start
  constraint coincident L1.end L2.start
  constraint coincident L103 A0.centre
  constraint midpoint L103 L104.start
  constraint midpoint L102 L104.end
  constraint midpoint L9 L105.start
  constraint midpoint L19 L105.end
  constraint coincident L103 A1.centre
  constraint equal A0 A1
  constraint symmetric A0 L104 A1
  constraint symmetric A0 L105 A2
  constraint symmetric L105 A1 A3
  measures "d40" diameter of A0
  measures "d41" distance of A0.centre A1.centre
extrude "Extrusion7" cut sketch "Skizze7" against normal blind 9.4 contours A0 | A1 | A2 | A3 bodies 3 4
sketch "Skizze8" plane through (0, 0, 1.8) normal (0, 0, -1) x (1, 0, 0)
  circle A0 centre (-2.8, -44) radius 1.7
  circle A1 centre (162.8, -44) radius 1.7
  circle A2 centre (-2.8, -20) radius 1.7
  circle A3 centre (162.8, -20) radius 1.7
  line L0 (4, 0) -> (0, -4)
  line L1 (0, -4) -> (0, -12)
  line L2 (0, -12) -> (-4, -12)
  line L3 (-4, -12) -> (-8, -16)
  line L4 (-8, -16) -> (-8, -48)
  line L5 (-8, -48) -> (-4, -52)
  line L6 (-4, -52) -> (0, -52)
  line L7 (0, -52) -> (0, -60)
  line L8 (0, -60) -> (4, -64)
  line L9 (4, -64) -> (156, -64)
  line L10 (156, -64) -> (160, -60)
  line L11 (160, -60) -> (160, -52)
  line L12 (160, -52) -> (164, -52)
  line L13 (164, -52) -> (168, -48)
  line L14 (168, -48) -> (168, -16)
  line L15 (168, -16) -> (164, -12)
  line L16 (164, -12) -> (160, -12)
  line L17 (160, -12) -> (160, -4)
  line L18 (160, -4) -> (156, 0)
  line L19 (156, 0) -> (4, 0)
  line L20 (155.2544, -62.2) -> (4.7456, -62.2)
  line L21 (4.7456, -62.2) -> (1.8, -59.2544)
  line L22 (1.8, -59.2544) -> (1.8, -4.7456)
  line L23 (1.8, -4.7456) -> (4.7456, -1.8)
  line L24 (4.7456, -1.8) -> (155.2544, -1.8)
  line L25 (155.2544, -1.8) -> (158.2, -4.7456)
  line L26 (158.2, -4.7456) -> (158.2, -59.2544)
  line L27 (158.2, -59.2544) -> (155.2544, -62.2)
  circle A4 centre (-2.8, -20) radius 2.4
  circle A5 centre (-2.8, -44) radius 2.4
  circle A6 centre (162.8, -44) radius 2.4
  circle A7 centre (162.8, -20) radius 2.4
  dimension "d44" = 4.8
  constraint concentric A2 A4
  constraint concentric A0 A5
  constraint concentric A1 A6
  constraint concentric A3 A7
  constraint equal A4 A7
  constraint equal A4 A5
  constraint equal A4 A6
  measures "d44" diameter of A4
extrude "Extrusion8" cut sketch "Skizze8" against normal blind 4.6 contours A4 | A5 | A6 | A7 bodies 3
chamfer "Fase3" distance 0.4 angle 45 4 edges at (-5.0376, 19.1321, 1.8) (-5.0376, 43.1321, 1.8) (160.5624, 43.1321, 1.8) (160.5624, 19.1321, 1.8) on bodies 3
chamfer "Fase4" distance 8 angle 45 2 edges at (0, 32, 7.6) (160, 32, 7.6) on bodies 3
ref_plane "Arbeitsebene3" through (80, 32, 20.9) normal (0, 0, 1) x (1, 0, 0)
mirror "Spiegeln1" about plane through (80, 32, 20.9) normal (0, 0, 1) of bodies 3 merged
sketch "Skizze9" plane through (0, 0, 40) normal (0, 0, 1) x (-1, 0, 0)
  circle A0 centre (-162.8, -20) radius 2.8
  circle A1 centre (-162.8, -44) radius 2.8
  circle A2 centre (2.8, -44) radius 2.8
  circle A3 centre (2.8, -20) radius 2.8
  line L0 (-155.2544, -62.2) -> (-158.2, -59.2544)
  line L1 (-158.2, -59.2544) -> (-158.2, -4.7456)
  line L2 (-158.2, -4.7456) -> (-155.2544, -1.8)
  line L3 (-155.2544, -1.8) -> (-4.7456, -1.8)
  line L4 (-4.7456, -1.8) -> (-1.8, -4.7456)
  line L5 (-1.8, -4.7456) -> (-1.8, -59.2544)
  line L6 (-1.8, -59.2544) -> (-4.7456, -62.2)
  line L7 (-4.7456, -62.2) -> (-155.2544, -62.2)
  line L8 (-4, -64) -> (0, -60)
  line L9 (0, -60) -> (0, -52)
  line L10 (0, -52) -> (4, -52)
  line L11 (4, -52) -> (8, -48)
  line L12 (8, -48) -> (8, -16)
  line L13 (8, -16) -> (4, -12)
  line L14 (4, -12) -> (0, -12)
  line L15 (0, -12) -> (0, -4)
  line L16 (0, -4) -> (-4, 0)
  line L17 (-4, 0) -> (-156, 0)
  line L18 (-156, 0) -> (-160, -4)
  line L19 (-160, -4) -> (-160, -12)
  line L20 (-160, -12) -> (-164, -12)
  line L21 (-164, -12) -> (-168, -16)
  line L22 (-168, -16) -> (-168, -48)
  line L23 (-168, -48) -> (-164, -52)
  line L24 (-164, -52) -> (-160, -52)
  line L25 (-160, -52) -> (-160, -60)
  line L26 (-160, -60) -> (-156, -64)
  line L27 (-156, -64) -> (-4, -64)
  circle A4 centre (2.8, -44) radius 1.7
  circle A5 centre (2.8, -20) radius 1.7
  circle A6 centre (-162.8, -44) radius 1.7
  circle A7 centre (-162.8, -20) radius 1.7
  dimension "d51" = 3.4
  constraint concentric A2 A4
  constraint concentric A3 A5
  constraint concentric A1 A6
  constraint concentric A0 A7
  constraint equal A4 A6
  constraint equal A4 A5
  constraint equal A4 A7
  measures "d51" diameter of A4
extrude "Extrusion9" add sketch "Skizze9" along normal blind 1.8 separate body contours A0 | A1 | A2 | A3 | L0 L1 L2 L3 L4 L5 L6 L7 | L8 L9 L10 L11 L12 L13 L14 L15 L16 L17 L18 L19 L20 L21 L22 L23 L24 L25 L26 L27 makes body 5
sketch "Skizze10" plane through (0, 0, 41.8) normal (0, 0, 1) x (-1, 0, 0)
  circle A0 centre (2.8, -20) radius 1.7
  circle A1 centre (2.8, -44) radius 1.7
  circle A2 centre (-162.8, -20) radius 1.7
  circle A3 centre (-162.8, -44) radius 1.7
  line L0 (-156, -64) -> (-4, -64)
  line L1 (-4, -64) -> (0, -60)
  line L2 (0, -60) -> (0, -52)
  line L3 (0, -52) -> (4, -52)
  line L4 (4, -52) -> (8, -48)
  line L5 (8, -48) -> (8, -16)
  line L6 (8, -16) -> (4, -12)
  line L7 (4, -12) -> (0, -12)
  line L8 (0, -12) -> (0, -4)
  line L9 (0, -4) -> (-4, 0)
  line L10 (-4, 0) -> (-156, 0)
  line L11 (-156, 0) -> (-160, -4)
  line L12 (-160, -4) -> (-160, -12)
  line L13 (-160, -12) -> (-164, -12)
  line L14 (-164, -12) -> (-168, -16)
  line L15 (-168, -16) -> (-168, -48)
  line L16 (-168, -48) -> (-164, -52)
  line L17 (-164, -52) -> (-160, -52)
  line L18 (-160, -52) -> (-160, -60)
  line L19 (-160, -60) -> (-156, -64)
  line L20 (8, -32) -> (-168, -32) construction
  line L21 (-80, -64) -> (-80, 0) construction
  line L22 (-67, -57) -> (-17, -57) construction
  line L23 (-17, -57) -> (-17, -7) construction
  line L24 (-17, -7) -> (-67, -7) construction
  line L25 (-67, -7) -> (-67, -57) construction
  line L26 (-67, -57) -> (-17, -7) construction
  line L27 (-17, -57) -> (-67, -7) construction
  circle A4 centre (-17, -7) radius 1.7
  circle A5 centre (-67, -57) radius 1.7
  circle A6 centre (-42, -32) radius 28
  circle A7 centre (-118, -32) radius 28
  circle A8 centre (-93, -7) radius 1.7
  circle A9 centre (-143, -57) radius 1.7
  circle A10 centre (-42, -32) radius 23
  circle A11 centre (-42, -32) radius 21
  circle A12 centre (-42, -32) radius 17
  circle A13 centre (-42, -32) radius 15
  circle A14 centre (-42, -32) radius 11
  line L28 (-14.0145, -32.9) -> (-19.0176, -32.9)
  line L29 (-21.0193, -32.9) -> (-25.0238, -32.9)
  line L30 (-27.027, -32.9) -> (-31.0369, -32.9)
  line L31 (-14.0145, -31.1) -> (-19.0176, -31.1)
  line L32 (-21.0193, -31.1) -> (-25.0238, -31.1)
  line L33 (-27.027, -31.1) -> (-31.0369, -31.1)
  line L34 (-41.1, -4.0145) -> (-41.1, -9.0176)
  line L35 (-41.1, -11.0193) -> (-41.1, -15.0238)
  line L36 (-42.9, -11.0193) -> (-42.9, -15.0238)
  line L37 (-41.1, -17.027) -> (-41.1, -21.0369)
  line L38 (-42.9, -17.027) -> (-42.9, -21.0369)
  line L39 (-42.9, -4.0145) -> (-42.9, -9.0176)
  line L40 (-69.9855, -31.1) -> (-64.9824, -31.1)
  line L41 (-62.9807, -31.1) -> (-58.9762, -31.1)
  line L42 (-62.9807, -32.9) -> (-58.9762, -32.9)
  line L43 (-56.973, -31.1) -> (-52.9631, -31.1)
  line L44 (-56.973, -32.9) -> (-52.9631, -32.9)
  line L45 (-69.9855, -32.9) -> (-64.9824, -32.9)
  line L46 (-42.9, -59.9855) -> (-42.9, -54.9824)
  line L47 (-42.9, -52.9807) -> (-42.9, -48.9762)
  line L48 (-41.1, -52.9807) -> (-41.1, -48.9762)
  line L49 (-42.9, -46.973) -> (-42.9, -42.9631)
  line L50 (-41.1, -46.973) -> (-41.1, -42.9631)
  line L51 (-41.1, -59.9855) -> (-41.1, -54.9824)
  line L52 (-118.9, -59.9855) -> (-118.9, -54.9824)
  circle A15 centre (-118, -32) radius 23
  circle A16 centre (-118, -32) radius 21
  line L53 (-118.9, -52.9807) -> (-118.9, -48.9762)
  line L54 (-117.1, -52.9807) -> (-117.1, -48.9762)
  line L55 (-117.1, -59.9855) -> (-117.1, -54.9824)
  circle A17 centre (-118, -32) radius 17
  circle A18 centre (-118, -32) radius 15
  line L56 (-118.9, -46.973) -> (-118.9, -42.9631)
  line L57 (-117.1, -46.973) -> (-117.1, -42.9631)
  circle A19 centre (-118, -32) radius 11
  line L58 (-132.973, -32.9) -> (-128.9631, -32.9)
  line L59 (-138.9807, -32.9) -> (-134.9762, -32.9)
  line L60 (-145.9855, -32.9) -> (-140.9824, -32.9)
  line L61 (-145.9855, -31.1) -> (-140.9824, -31.1)
  line L62 (-138.9807, -31.1) -> (-134.9762, -31.1)
  line L63 (-132.973, -31.1) -> (-128.9631, -31.1)
  line L64 (-118.9, -17.027) -> (-118.9, -21.0369)
  line L65 (-118.9, -11.0193) -> (-118.9, -15.0238)
  line L66 (-118.9, -4.0145) -> (-118.9, -9.0176)
  line L67 (-117.1, -4.0145) -> (-117.1, -9.0176)
  line L68 (-117.1, -11.0193) -> (-117.1, -15.0238)
  line L69 (-117.1, -17.027) -> (-117.1, -21.0369)
  line L70 (-103.027, -31.1) -> (-107.0369, -31.1)
  line L71 (-103.027, -32.9) -> (-107.0369, -32.9)
  line L72 (-97.0193, -32.9) -> (-101.0238, -32.9)
  line L73 (-97.0193, -31.1) -> (-101.0238, -31.1)
  line L74 (-90.0145, -32.9) -> (-95.0176, -32.9)
  line L75 (-90.0145, -31.1) -> (-95.0176, -31.1)
  line L76 (-93, -7) -> (-143, -7) construction
  line L77 (-143, -7) -> (-143, -57) construction
  line L78 (-143, -57) -> (-93, -57) construction
  line L79 (-93, -57) -> (-93, -7) construction
  line L80 (-93, -7) -> (-143, -57) construction
  line L81 (-143, -7) -> (-93, -57) construction
  point P0 (-42, -32)
  point P1 (-118, -32)
  dimension "d54" = 50
  dimension "d55" = 50
  dimension "d57" = 38
  dimension "d58" = 56
  dimension "d59" = 46
  dimension "d60" = 42
  dimension "d61" = 34
  dimension "d62" = 30
  dimension "d63" = 22
  dimension "d64" = 0.9
  dimension "d66" = 360
  dimension "d77" = 3.4
  dimension "d78" = 3.4
  dimension "d79" = 50
  dimension "d80" = 50
  constraint midpoint L5 L20.start
  constraint midpoint L15 L20.end
  constraint midpoint L0 L21.start
  constraint midpoint L10 L21.end
  constraint horizontal L22
  constraint perpendicular L22 L23
  constraint parallel L22 L24
  constraint parallel L23 L25
  constraint coincident L26 P0
  constraint coincident L27 P0
  constraint coincident L20 P0
  constraint coincident L23.end L24.start
  constraint coincident L22.start L25.end
  constraint coincident P0 A6.centre
  constraint symmetric L21 A6 A7
  constraint concentric A11 A12
  constraint concentric A6 A13
  constraint concentric A6 A14
  constraint coincident A6 L28.start
  constraint coincident A10 L28.end
  constraint perpendicular L23 L28
  constraint coincident A11 L29.start
  constraint coincident A12 L29.end
  constraint parallel L28 L29
  constraint coincident A13 L30.start
  constraint coincident A14 L30.end
  constraint parallel L29 L30
  constraint collinear L28 L29
  constraint collinear L28 L30
  constraint symmetric L20 L28.start L31.start
  constraint symmetric L20 L28.end L31.end
  constraint symmetric L20 L29.start L32.start
  constraint symmetric L20 L29.end L32.end
  constraint symmetric L20 L30.start L33.start
  constraint symmetric L20 L30.end L33.end
  constraint symmetric L21 A10 A15
  constraint symmetric L21 A11 A16
  constraint symmetric L21 A12 A17
  constraint symmetric L21 A13 A18
  constraint symmetric L21 A14 A19
  constraint symmetric L21 L28.start L60.start
  constraint symmetric L21 L28.end L60.end
  constraint symmetric L21 L29.start L59.start
  constraint symmetric L21 L29.end L59.end
  constraint symmetric L21 L30.start L58.start
  constraint symmetric L21 L30.end L58.end
  constraint symmetric L21 L31.start L61.start
  constraint symmetric L21 L31.end L61.end
  constraint symmetric L21 L32.start L62.start
  constraint symmetric L21 L32.end L62.end
  constraint symmetric L21 L33.start L63.start
  constraint symmetric L21 L33.end L63.end
  constraint symmetric L21 L34.start L66.start
  constraint symmetric L21 L34.end L66.end
  constraint symmetric L21 L35.start L65.start
  constraint symmetric L21 L35.end L65.end
  constraint symmetric L21 L36.start L68.start
  constraint symmetric L21 L36.end L68.end
  constraint symmetric L21 L37.start L64.start
  constraint symmetric L21 L37.end L64.end
  constraint symmetric L21 L38.start L69.start
  constraint symmetric L21 L38.end L69.end
  constraint symmetric L21 L39.start L67.start
  constraint symmetric L21 L39.end L67.end
  constraint symmetric L21 L40.start L75.start
  constraint symmetric L21 L40.end L75.end
  constraint symmetric L21 L41.start L73.start
  constraint symmetric L21 L41.end L73.end
  constraint symmetric L21 L42.start L72.start
  constraint symmetric L21 L42.end L72.end
  constraint symmetric L21 L43.start L70.start
  constraint symmetric L21 L43.end L70.end
  constraint symmetric L21 L44.start L71.start
  constraint symmetric L21 L44.end L71.end
  constraint symmetric L21 L45.start L74.start
  constraint symmetric L21 L45.end L74.end
  constraint symmetric L21 L46.start L55.start
  constraint symmetric L21 L46.end L55.end
  constraint symmetric L21 L47.start L54.start
  constraint symmetric L21 L47.end L54.end
  constraint symmetric L21 L48.start L53.start
  constraint symmetric L21 L48.end L53.end
  constraint symmetric L21 L49.start L57.start
  constraint symmetric L21 L49.end L57.end
  constraint symmetric L21 L50.start L56.start
  constraint symmetric L21 L50.end L56.end
  constraint symmetric L21 L51.start L52.start
  constraint symmetric L21 L51.end L52.end
  constraint equal A4 A5
  constraint horizontal L76
  constraint perpendicular L76 L77
  constraint parallel L76 L78
  constraint parallel L77 L79
  constraint coincident A8.centre L76.start
  constraint coincident L80 P1
  constraint coincident L81 P1
  constraint coincident P1 A7.centre
  measures "d54" distance of L23.end L24.end
  measures "d55" distance of L22.end L23.end
  measures "d57" distance of L21 P0
  measures "d58" diameter of A6
  measures "d59" diameter of A10
  measures "d60" diameter of A11
  measures "d61" diameter of A12
  measures "d62" diameter of A13
  measures "d63" diameter of A14
  measures "d64" distance of L20 L28
  measures "d77" diameter of A5
  measures "d78" diameter of A8
  measures "d79" distance of A9.centre L78.end
  measures "d80" distance of A8.centre L78.end
extrude "Extrusion10" cut sketch "Skizze10" against normal blind 1.8 contours A4 | A5 | A6 A10 L31 L34 | A6 A10 L28 L51 | A6 A10 L39 L40 | A6 A10 L45 L46 | A7 A15 L67 L75 | A7 A15 L55 L74 | A7 A15 L61 L66 | A7 L52 A15 L60 | A8 | A9 | A11 A12 L32 L35 | A11 A12 L29 L48 | A11 A12 L36 L41 | A11 A12 L42 L47 | A13 A14 L33 L37 | A13 A14 L30 L50 | A13 A14 L38 L43 | A13 A14 L44 L49 | A16 A17 L68 L73 | A16 L54 A17 L72 | A16 A17 L62 L65 | A16 L53 A17 L59 | A18 A19 L69 L70 | A18 L57 A19 L71 | A18 A19 L63 L64 | A18 L56 A19 L58 bodies 5
copy_body "Körper->Berechn1" bodies 3 removing the originals makes body 6 in component "Main Body"
copy_body "Körper->Berechn2" bodies 4 removing the originals makes body 7 in component "Inside Cover"
copy_body "Körper->Berechn3" bodies 5 removing the originals makes body 8 in component "Back Cover"
sketch "Skizze11" plane through (0, 0, 0) normal (0, -1, 0) x (1, 0, 0)
  line L0 (4, 1.8) -> (156, 1.8)
  line L1 (156, 1.8) -> (156, 40)
  line L2 (156, 40) -> (4, 40)
  line L3 (4, 40) -> (4, 1.8)
  line L4 (80, 40) -> (80, 1.8) construction
  line L5 (78.5, 37) -> (81.5, 37)
  line L6 (81.5, 37) -> (81.5, 40)
  line L7 (81.5, 40) -> (78.5, 40)
  line L8 (78.5, 40) -> (78.5, 37)
  dimension "d81" = 3
  dimension "d82" = 3
  constraint midpoint L2 L4.start
  constraint midpoint L0 L4.end
  constraint horizontal L5
  constraint vertical L6
  constraint horizontal L7
  constraint vertical L8
  constraint coincident L2 L6.end
  constraint symmetric L4 L6 L8
  measures "d81" distance of L5.end L6.end
  measures "d82" distance of L5.start L5.end
sketch "Skizze12" plane through (0, 0, 40) normal (0, 0, 1) x (-1, 0, 0)
  line L0 (-156, 0) -> (-160, -4)
  line L1 (-160, -4) -> (-160, -12)
  line L2 (-160, -12) -> (-164, -12)
  line L3 (-164, -12) -> (-168, -16)
  line L4 (-168, -16) -> (-168, -48)
  line L5 (-168, -48) -> (-164, -52)
  line L6 (-164, -52) -> (-160, -52)
  line L7 (-160, -52) -> (-160, -60)
  line L8 (-160, -60) -> (-156, -64)
  line L9 (-156, -64) -> (-4, -64)
  line L10 (-4, -64) -> (0, -60)
  line L11 (0, -60) -> (0, -52)
  line L12 (0, -52) -> (4, -52)
  line L13 (4, -52) -> (8, -48)
  line L14 (8, -48) -> (8, -16)
  line L15 (8, -16) -> (4, -12)
  line L16 (4, -12) -> (0, -12)
  line L17 (0, -12) -> (0, -4)
  line L18 (0, -4) -> (-4, 0)
  line L19 (-4, 0) -> (-156, 0)
  line L20 (-4.7456, -1.8) -> (-1.8, -4.7456)
  line L21 (-1.8, -4.7456) -> (-1.8, -59.2544)
  line L22 (-1.8, -59.2544) -> (-4.7456, -62.2)
  line L23 (-4.7456, -62.2) -> (-155.2544, -62.2)
  line L24 (-155.2544, -62.2) -> (-158.2, -59.2544)
  line L25 (-158.2, -59.2544) -> (-158.2, -4.7456)
  line L26 (-158.2, -4.7456) -> (-155.2544, -1.8)
  line L27 (-155.2544, -1.8) -> (-4.7456, -1.8)
  circle A0 centre (-162.8, -20) radius 2.8
  circle A1 centre (-162.8, -44) radius 2.8
  circle A2 centre (2.8, -44) radius 2.8
  circle A3 centre (2.8, -20) radius 2.8
  line L28 (-78.5, -2.8) -> (-5.1598, -2.8)
  line L29 (-5.1598, -2.8) -> (-2.8, -5.1598)
  line L30 (-2.8, -5.1598) -> (-2.8, -58.8402)
  line L31 (-2.8, -58.8402) -> (-5.1598, -61.2)
  line L32 (-5.1598, -61.2) -> (-154.8402, -61.2)
  line L33 (-154.8402, -61.2) -> (-157.2, -58.8402)
  line L34 (-157.2, -58.8402) -> (-157.2, -5.1598)
  line L35 (-157.2, -5.1598) -> (-154.8402, -2.8)
  line L36 (-154.8402, -2.8) -> (-81.5, -2.8)
  line L37 (-78.5, -2.8) -> (-81.5, -2.8)
  constraint parallel L20 L29
  constraint parallel L21 L30
  constraint parallel L22 L31
  constraint parallel L23 L32
  constraint parallel L24 L33
  constraint parallel L25 L34
  constraint parallel L26 L35
  constraint parallel L27 L36
extrude "Extrusion11" add sketch "Skizze12" along normal blind 1 from surface at -16 separate body contours L28 L29 L30 L31 L32 L33 L34 L35 L36 L37 makes body 9
copy_body "Körper->Berechn4" bodies 9 removing the originals makes body 10 in component "Fan Protection"